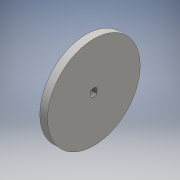
# Autodesk Inventor part: wheel small
Saved by Autodesk Inventor 2016 (Build 200138000, 138)
## iProperties
Created: 2015-09-14
Part Number: wheel small
Material: Generic
Document SubType Name: Modeling
Designer: Hulbert Office
Density: 1 g/cm^3
Appearance: Default
Author: Hulbert Office
Autodesk Inventor part; units mm, degrees
ref_plane "YZ Plane" through (0, 0, 0) normal (1, 0, 0) x (0, 1, 0)
ref_plane "XZ Plane" through (0, 0, 0) normal (0, 1, 0) x (-1, 0, 0)
ref_plane "XY Plane" through (0, 0, 0) normal (0, 0, 1) x (1, 0, 0)
sketch "Sketch1" plane through (0, 0, 0) normal (1, 0, 0) x (0, 1, 0)
  circle A0 centre (0, 0) radius 24
  circle A1 centre (0, 0) radius 2
  dimension "d0" = 48
  dimension "d1" = 4
  constraints: 2 centre point, 2 coincident
  measures "d0" diameter of A0
  measures "d1" diameter of A1
extrude "Extrusion1" add sketch "Sketch1" along normal blind 4
sketch "Sketch3" plane through (4, 0, 0) normal (1, 0, 0) x (0, 0, -1)
  circle A0 centre (0, 0) radius 2 projected
  line L0 (0, -2) -> (0, 1.5)
  line L1 (0, 1.5) -> (1.3229, 1.5)
  line L2 (0, 1.5) -> (-1.3229, 1.5)
  dimension "d7" = 3.5
  constraints: 6 end point, 3 point on circle, 1 perpendicular, 1 point on line, 1 vertical
  measures "d7" distance of L0.start L0.end
extrude "Extrusion3" add sketch "Sketch3" against normal blind 4 contours L1 L2 A0
body "Solid1"
